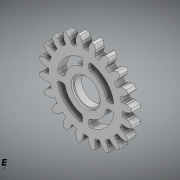
# Autodesk Inventor part: m2z20
Saved by Autodesk Inventor 2020 (Build 240168000, 168)
## iProperties
Created: 2019-12-19
Part Number: m2z20
Material: 一般
Document SubType Name: Modeling
Designer: hamaa
Density: 1 g/cm^3
Appearance: 既定
Author: hamaa
Autodesk Inventor part; units mm, degrees
(part 1 of 2)
ref_plane "YZ Plane" through (0, 0, 0) normal (1, 0, 0) x (0, 1, 0)
ref_plane "XZ Plane" through (0, 0, 0) normal (0, 1, 0) x (-1, 0, 0)
ref_plane "XY Plane" through (0, 0, 0) normal (0, 0, 1) x (1, 0, 0)
sketch "スケッチ1" plane through (0, 0, 0) normal (0, 0, 1) x (1, 0, 0)
  arc A0 (149.7476, 124.0441) -> (149.6952, 123.7559) centre (151.6276, 123.5535) ccw
  arc A1 (150.1104, 125.0278) -> (149.7476, 124.0441) centre (154.9305, 122.6916) ccw
  arc A2 (151.2536, 126.8271) -> (150.1104, 125.0278) centre (158.4906, 120.9661) ccw
  arc A3 (143.8017, 123.4975) -> (143.8409, 123.2073) centre (145.7412, 123.6119) ccw
  arc A4 (143.8427, 124.5452) -> (143.8017, 123.4975) centre (149.1488, 123.8129) ccw
  arc A5 (144.3739, 126.6097) -> (143.8427, 124.5452) centre (153.0679, 123.272) ccw
  arc A6 (138.3156, 121.1404) -> (138.4426, 120.8764) centre (140.1248, 121.8485) ccw
  arc A7 (138.0309, 122.1494) -> (138.3156, 121.1404) centre (143.3036, 123.0926) ccw
  arc A8 (137.8981, 124.2771) -> (138.0309, 122.1494) centre (147.198, 123.7893) ccw
  arc A9 (133.8264, 117.2033) -> (134.0288, 116.9915) centre (135.3283, 118.4358) ccw
  arc A10 (133.2438, 118.0749) -> (133.8264, 117.2033) centre (137.967, 120.6013) ccw
  arc A11 (132.4601, 120.0574) -> (133.2438, 118.0749) centre (141.4555, 122.4673) ccw
  arc A12 (130.7736, 112.0716) -> (131.0315, 111.9328) centre (131.8211, 113.708) ccw
  arc A13 (129.9502, 112.7206) -> (130.7736, 112.0716) centre (133.6615, 116.5829) ccw
  arc A14 (128.5922, 114.3639) -> (129.9502, 112.7206) centre (136.4027, 119.4356) ccw
  arc A15 (129.456, 106.2478) -> (129.7442, 106.1954) centre (129.9466, 108.1277) ccw
  arc A16 (128.4723, 106.6105) -> (129.456, 106.2478) centre (130.8085, 111.4307) ccw
  arc A17 (126.673, 107.7538) -> (128.4723, 106.6105) centre (132.5339, 114.9908) ccw
  arc A18 (130.0025, 100.3018) -> (130.2928, 100.341) centre (129.8882, 102.2413) ccw
  arc A19 (128.9549, 100.3428) -> (130.0025, 100.3018) centre (129.6872, 105.649) ccw
  arc A20 (126.8903, 100.8741) -> (128.9549, 100.3428) centre (130.2281, 109.568) ccw
  arc A21 (132.3597, 94.8158) -> (132.6237, 94.9428) centre (131.6516, 96.625) ccw
  arc A22 (131.3507, 94.531) -> (132.3597, 94.8158) centre (130.4075, 99.8038) ccw
  arc A23 (129.223, 94.3983) -> (131.3507, 94.531) centre (129.7108, 103.6981) ccw
  arc A24 (136.2968, 90.3266) -> (136.5086, 90.529) centre (135.0643, 91.8285) ccw
  arc A25 (135.4252, 89.744) -> (136.2968, 90.3266) centre (132.8988, 94.4672) ccw
  arc A26 (133.4426, 88.9603) -> (135.4252, 89.744) centre (131.0328, 97.9557) ccw
  arc A27 (141.4285, 87.2738) -> (141.5673, 87.5317) centre (139.7921, 88.3213) ccw
  arc A28 (140.7795, 86.4504) -> (141.4285, 87.2738) centre (136.9172, 90.1617) ccw
  arc A29 (139.1362, 85.0923) -> (140.7795, 86.4504) centre (134.0645, 92.9028) ccw
  arc A30 (147.2523, 85.9562) -> (147.3047, 86.2444) centre (145.3724, 86.4467) ccw
  arc A31 (146.8896, 84.9725) -> (147.2523, 85.9562) centre (142.0694, 87.3087) ccw
  arc A32 (145.7463, 83.1731) -> (146.8896, 84.9725) centre (138.5093, 89.0341) ccw
  arc A33 (153.1983, 86.5027) -> (153.159, 86.793) centre (151.2588, 86.3883) ccw
  arc A34 (153.1573, 85.4551) -> (153.1983, 86.5027) centre (147.8511, 86.1874) ccw
  arc A35 (152.626, 83.3905) -> (153.1573, 85.4551) centre (143.9321, 86.7283) ccw
  arc A36 (158.6843, 88.8599) -> (158.5573, 89.1238) centre (156.8751, 88.1518) ccw
  arc A37 (158.9691, 87.8509) -> (158.6843, 88.8599) centre (153.6963, 86.9076) ccw
  arc A38 (159.1018, 85.7232) -> (158.9691, 87.8509) centre (149.8019, 86.211) ccw
  arc A39 (163.1735, 92.797) -> (162.9711, 93.0088) centre (161.6716, 91.5644) ccw
  arc A40 (163.7561, 91.9254) -> (163.1735, 92.797) centre (159.0329, 89.3989) ccw
  arc A41 (164.5398, 89.9428) -> (163.7561, 91.9254) centre (155.5444, 87.5329) ccw
  arc A42 (166.2263, 97.9286) -> (165.9684, 98.0675) centre (165.1788, 96.2923) ccw
  arc A43 (167.0497, 97.2797) -> (166.2263, 97.9286) centre (163.3384, 93.4173) ccw
  arc A44 (168.4077, 95.6364) -> (167.0497, 97.2797) centre (160.5973, 90.5647) ccw
  arc A45 (167.5439, 103.7525) -> (167.2557, 103.8049) centre (167.0533, 101.8725) ccw
  arc A46 (168.5276, 103.3897) -> (167.5439, 103.7525) centre (166.1914, 98.5696) ccw
  arc A47 (170.327, 102.2465) -> (168.5276, 103.3897) centre (164.466, 95.0095) ccw
  arc A48 (166.9974, 109.6984) -> (166.7071, 109.6592) centre (167.1118, 107.7589) ccw
  arc A49 (168.045, 109.6574) -> (166.9974, 109.6984) centre (167.3127, 104.3513) ccw
  arc A50 (170.1096, 109.1262) -> (168.045, 109.6574) centre (166.7718, 100.4322) ccw
  arc A51 (164.6402, 115.1845) -> (164.3763, 115.0575) centre (165.3483, 113.3753) ccw
  arc A52 (165.6492, 115.4692) -> (164.6402, 115.1845) centre (166.5924, 110.1965) ccw
  arc A53 (167.7769, 115.602) -> (165.6492, 115.4692) centre (167.2891, 106.3021) ccw
  arc A54 (160.7031, 119.6736) -> (160.4913, 119.4713) centre (161.9356, 118.1718) ccw
  arc A55 (161.5747, 120.2563) -> (160.7031, 119.6736) centre (164.1012, 115.533) ccw
  arc A56 (163.5573, 121.04) -> (161.5747, 120.2563) centre (165.9672, 112.0445) ccw
  arc A57 (155.5715, 122.7265) -> (155.4326, 122.4686) centre (157.2078, 121.679) ccw
  arc A58 (156.2204, 123.5499) -> (155.5715, 122.7265) centre (160.0827, 119.8386) ccw
  arc A59 (157.8637, 124.9079) -> (156.2204, 123.5499) centre (162.9354, 117.0974) ccw
  arc A60 (147.3047, 123.7559) -> (147.2523, 124.0441) centre (145.3724, 123.5535) ccw
  arc A61 (147.2523, 124.0441) -> (146.8896, 125.0278) centre (142.0694, 122.6916) ccw
  arc A62 (146.8896, 125.0278) -> (145.7463, 126.8271) centre (138.5093, 120.9661) ccw
  arc A63 (141.5673, 122.4686) -> (141.4285, 122.7265) centre (139.7921, 121.679) ccw
  arc A64 (141.4285, 122.7265) -> (140.7795, 123.5499) centre (136.9172, 119.8386) ccw
  arc A65 (140.7795, 123.5499) -> (139.1362, 124.9079) centre (134.0645, 117.0974) ccw
  arc A66 (136.5086, 119.4713) -> (136.2968, 119.6736) centre (135.0643, 118.1718) ccw
  arc A67 (136.2968, 119.6736) -> (135.4252, 120.2563) centre (132.8988, 115.533) ccw
  arc A68 (135.4252, 120.2563) -> (133.4426, 121.04) centre (131.0328, 112.0445) ccw
  arc A69 (132.6237, 115.0575) -> (132.3597, 115.1845) centre (131.6516, 113.3753) ccw
  arc A70 (132.3597, 115.1845) -> (131.3507, 115.4692) centre (130.4075, 110.1965) ccw
  arc A71 (131.3507, 115.4692) -> (129.223, 115.602) centre (129.7108, 106.3021) ccw
  arc A72 (130.2928, 109.6592) -> (130.0025, 109.6984) centre (129.8882, 107.7589) ccw
  arc A73 (130.0025, 109.6984) -> (128.9549, 109.6574) centre (129.6872, 104.3513) ccw
  arc A74 (128.9549, 109.6574) -> (126.8903, 109.1262) centre (130.2281, 100.4322) ccw
  arc A75 (129.7442, 103.8049) -> (129.456, 103.7525) centre (129.9466, 101.8725) ccw
  arc A76 (129.456, 103.7525) -> (128.4723, 103.3897) centre (130.8085, 98.5696) ccw
  arc A77 (128.4723, 103.3897) -> (126.673, 102.2465) centre (132.5339, 95.0095) ccw
  arc A78 (131.0315, 98.0675) -> (130.7736, 97.9286) centre (131.8211, 96.2923) ccw
  arc A79 (130.7736, 97.9286) -> (129.9502, 97.2797) centre (133.6615, 93.4173) ccw
  arc A80 (129.9502, 97.2797) -> (128.5922, 95.6364) centre (136.4027, 90.5647) ccw
  arc A81 (134.0288, 93.0088) -> (133.8264, 92.797) centre (135.3283, 91.5644) ccw
  arc A82 (133.8264, 92.797) -> (133.2438, 91.9254) centre (137.967, 89.3989) ccw
  arc A83 (133.2438, 91.9254) -> (132.4601, 89.9428) centre (141.4555, 87.5329) ccw
  arc A84 (138.4426, 89.1238) -> (138.3156, 88.8599) centre (140.1248, 88.1518) ccw
  arc A85 (138.3156, 88.8599) -> (138.0309, 87.8509) centre (143.3036, 86.9076) ccw
  arc A86 (138.0309, 87.8509) -> (137.8981, 85.7232) centre (147.198, 86.211) ccw
  arc A87 (143.8409, 86.793) -> (143.8017, 86.5027) centre (145.7412, 86.3883) ccw
  arc A88 (143.8017, 86.5027) -> (143.8427, 85.4551) centre (149.1488, 86.1874) ccw
  arc A89 (143.8427, 85.4551) -> (144.3739, 83.3905) centre (153.0679, 86.7283) ccw
  arc A90 (149.6952, 86.2444) -> (149.7476, 85.9562) centre (151.6276, 86.4467) ccw
  arc A91 (149.7476, 85.9562) -> (150.1104, 84.9725) centre (154.9305, 87.3087) ccw
  arc A92 (150.1104, 84.9725) -> (151.2536, 83.1731) centre (158.4906, 89.0341) ccw
  arc A93 (155.4326, 87.5317) -> (155.5715, 87.2738) centre (157.2078, 88.3213) ccw
  arc A94 (155.5715, 87.2738) -> (156.2204, 86.4504) centre (160.0827, 90.1617) ccw
  arc A95 (156.2204, 86.4504) -> (157.8637, 85.0923) centre (162.9354, 92.9028) ccw
  arc A96 (160.4913, 90.529) -> (160.7031, 90.3266) centre (161.9356, 91.8285) ccw
  arc A97 (160.7031, 90.3266) -> (161.5747, 89.744) centre (164.1012, 94.4672) ccw
  arc A98 (161.5747, 89.744) -> (163.5573, 88.9603) centre (165.9672, 97.9557) ccw
  arc A99 (164.3763, 94.9428) -> (164.6402, 94.8158) centre (165.3483, 96.625) ccw
  arc A100 (164.6402, 94.8158) -> (165.6492, 94.531) centre (166.5924, 99.8038) ccw
  arc A101 (165.6492, 94.531) -> (167.7769, 94.3983) centre (167.2891, 103.6981) ccw
  arc A102 (166.7071, 100.341) -> (166.9974, 100.3018) centre (167.1118, 102.2413) ccw
  arc A103 (166.9974, 100.3018) -> (168.045, 100.3428) centre (167.3127, 105.649) ccw
  arc A104 (168.045, 100.3428) -> (170.1096, 100.8741) centre (166.7718, 109.568) ccw
  arc A105 (167.2557, 106.1954) -> (167.5439, 106.2478) centre (167.0533, 108.1277) ccw
  arc A106 (167.5439, 106.2478) -> (168.5276, 106.6105) centre (166.1914, 111.4307) ccw
  arc A107 (168.5276, 106.6105) -> (170.327, 107.7538) centre (164.466, 114.9908) ccw
  arc A108 (165.9684, 111.9328) -> (166.2263, 112.0716) centre (165.1788, 113.708) ccw
  arc A109 (166.2263, 112.0716) -> (167.0497, 112.7206) centre (163.3384, 116.5829) ccw
  arc A110 (167.0497, 112.7206) -> (168.4077, 114.3639) centre (160.5973, 119.4356) ccw
  arc A111 (162.9711, 116.9915) -> (163.1735, 117.2033) centre (161.6716, 118.4358) ccw
  arc A112 (163.1735, 117.2033) -> (163.7561, 118.0749) centre (159.0329, 120.6013) ccw
  arc A113 (163.7561, 118.0749) -> (164.5398, 120.0574) centre (155.5444, 122.4673) ccw
  arc A114 (158.5573, 120.8764) -> (158.6843, 121.1404) centre (156.8751, 121.8485) ccw
  arc A115 (158.6843, 121.1404) -> (158.9691, 122.1494) centre (153.6963, 123.0926) ccw
  arc A116 (158.9691, 122.1494) -> (159.1018, 124.2771) centre (149.8019, 123.7893) ccw
  arc A117 (153.159, 123.2073) -> (153.1983, 123.4975) centre (151.2588, 123.6119) ccw
  arc A118 (153.1983, 123.4975) -> (153.1573, 124.5452) centre (147.8511, 123.8129) ccw
  arc A119 (153.1573, 124.5452) -> (152.626, 126.6097) centre (143.9321, 123.272) ccw
  arc A120 (149.613, 122.4647) -> (147.387, 122.4647) centre (148.5, 105.0001) ccw
  arc A121 (144.1616, 121.9539) -> (142.0446, 121.266) centre (148.5, 105.0001) ccw
  arc A122 (139.135, 119.7835) -> (137.3341, 118.4751) centre (148.5, 105.0001) ccw
  arc A123 (135.025, 116.166) -> (133.7166, 114.3651) centre (148.5, 105.0001) ccw
  arc A124 (132.2341, 111.4555) -> (131.5462, 109.3385) centre (148.5, 105.0001) ccw
  arc A125 (131.0354, 106.1131) -> (131.0354, 103.8871) centre (148.5, 105.0001) ccw
  arc A126 (131.5462, 100.6618) -> (132.2341, 98.5448) centre (148.5, 105.0001) ccw
  arc A127 (133.7166, 95.6351) -> (135.025, 93.8343) centre (148.5, 105.0001) ccw
  arc A128 (137.3341, 91.5252) -> (139.135, 90.2168) centre (148.5, 105.0001) ccw
  arc A129 (142.0446, 88.7343) -> (144.1616, 88.0464) centre (148.5, 105.0001) ccw
  arc A130 (147.387, 87.5356) -> (149.613, 87.5356) centre (148.5, 105.0001) ccw
  arc A131 (152.8383, 88.0464) -> (154.9553, 88.7343) centre (148.5, 105.0001) ccw
  arc A132 (157.8649, 90.2168) -> (159.6658, 91.5252) centre (148.5, 105.0001) ccw
  arc A133 (161.9749, 93.8343) -> (163.2833, 95.6351) centre (148.5, 105.0001) ccw
  arc A134 (164.7658, 98.5448) -> (165.4537, 100.6618) centre (148.5, 105.0001) ccw
  arc A135 (165.9645, 103.8871) -> (165.9645, 106.1131) centre (148.5, 105.0001) ccw
  arc A136 (165.4537, 109.3385) -> (164.7658, 111.4555) centre (148.5, 105.0001) ccw
  arc A137 (163.2833, 114.3651) -> (161.9749, 116.166) centre (148.5, 105.0001) ccw
  arc A138 (159.6658, 118.4751) -> (157.8649, 119.7835) centre (148.5, 105.0001) ccw
  arc A139 (154.9553, 121.266) -> (152.8383, 121.9539) centre (148.5, 105.0001) ccw
  arc A140 (145.7463, 126.8271) -> (144.3739, 126.6097) centre (148.5, 105.0001) ccw
  arc A141 (139.1362, 124.9079) -> (137.8981, 124.2771) centre (148.5, 105.0001) ccw
  arc A142 (133.4426, 121.04) -> (132.4601, 120.0574) centre (148.5, 105.0001) ccw
  arc A143 (129.223, 115.602) -> (128.5922, 114.3639) centre (148.5, 105.0001) ccw
  arc A144 (126.8903, 109.1262) -> (126.673, 107.7538) centre (148.5, 105.0001) ccw
  arc A145 (126.673, 102.2465) -> (126.8903, 100.8741) centre (148.5, 105.0001) ccw
  arc A146 (128.5922, 95.6364) -> (129.223, 94.3983) centre (148.5, 105.0001) ccw
  arc A147 (132.4601, 89.9428) -> (133.4426, 88.9603) centre (148.5, 105.0001) ccw
  arc A148 (137.8981, 85.7232) -> (139.1362, 85.0923) centre (148.5, 105.0001) ccw
  arc A149 (144.3739, 83.3905) -> (145.7463, 83.1731) centre (148.5, 105.0001) ccw
  arc A150 (151.2536, 83.1731) -> (152.626, 83.3905) centre (148.5, 105.0001) ccw
  arc A151 (157.8637, 85.0923) -> (159.1018, 85.7232) centre (148.5, 105.0001) ccw
  arc A152 (163.5573, 88.9603) -> (164.5398, 89.9428) centre (148.5, 105.0001) ccw
  arc A153 (167.7769, 94.3983) -> (168.4077, 95.6364) centre (148.5, 105.0001) ccw
  arc A154 (170.1096, 100.8741) -> (170.327, 102.2465) centre (148.5, 105.0001) ccw
  arc A155 (170.327, 107.7538) -> (170.1096, 109.1262) centre (148.5, 105.0001) ccw
  arc A156 (168.4077, 114.3639) -> (167.7769, 115.602) centre (148.5, 105.0001) ccw
  arc A157 (164.5398, 120.0574) -> (163.5573, 121.04) centre (148.5, 105.0001) ccw
  arc A158 (159.1018, 124.2771) -> (157.8637, 124.9079) centre (148.5, 105.0001) ccw
  arc A159 (152.626, 126.6097) -> (151.2536, 126.8271) centre (148.5, 105.0001) ccw
  line L0 (149.613, 122.4647) -> (149.6952, 123.7559)
  line L1 (144.1616, 121.9539) -> (143.8409, 123.2073)
  line L2 (139.135, 119.7835) -> (138.4426, 120.8764)
  line L3 (135.025, 116.166) -> (134.0288, 116.9915)
  line L4 (132.2341, 111.4555) -> (131.0315, 111.9328)
  line L5 (131.0354, 106.1131) -> (129.7442, 106.1954)
  line L6 (131.5462, 100.6618) -> (130.2928, 100.341)
  line L7 (133.7166, 95.6351) -> (132.6237, 94.9428)
  line L8 (137.3341, 91.5252) -> (136.5086, 90.529)
  line L9 (142.0446, 88.7343) -> (141.5673, 87.5317)
  line L10 (147.387, 87.5356) -> (147.3047, 86.2444)
  line L11 (152.8383, 88.0464) -> (153.159, 86.793)
  line L12 (157.8649, 90.2168) -> (158.5573, 89.1238)
  line L13 (161.9749, 93.8343) -> (162.9711, 93.0088)
  line L14 (164.7658, 98.5448) -> (165.9684, 98.0675)
  line L15 (165.9645, 103.8871) -> (167.2557, 103.8049)
  line L16 (165.4537, 109.3385) -> (166.7071, 109.6592)
  line L17 (163.2833, 114.3651) -> (164.3763, 115.0575)
  line L18 (159.6658, 118.4751) -> (160.4913, 119.4713)
  line L19 (154.9553, 121.266) -> (155.4326, 122.4686)
  line L20 (147.387, 122.4647) -> (147.3047, 123.7559)
  line L21 (142.0446, 121.266) -> (141.5673, 122.4686)
  line L22 (137.3341, 118.4751) -> (136.5086, 119.4713)
  line L23 (133.7166, 114.3651) -> (132.6237, 115.0575)
  line L24 (131.5462, 109.3385) -> (130.2928, 109.6592)
  line L25 (131.0354, 103.8871) -> (129.7442, 103.8049)
  line L26 (132.2341, 98.5448) -> (131.0315, 98.0675)
  line L27 (135.025, 93.8343) -> (134.0288, 93.0088)
  line L28 (139.135, 90.2168) -> (138.4426, 89.1238)
  line L29 (144.1616, 88.0464) -> (143.8409, 86.793)
  line L30 (149.613, 87.5356) -> (149.6952, 86.2444)
  line L31 (154.9553, 88.7343) -> (155.4326, 87.5317)
  line L32 (159.6658, 91.5252) -> (160.4913, 90.529)
  line L33 (163.2833, 95.6351) -> (164.3763, 94.9428)
  line L34 (165.4537, 100.6618) -> (166.7071, 100.341)
  line L35 (165.9645, 106.1131) -> (167.2557, 106.1954)
  line L36 (164.7658, 111.4555) -> (165.9684, 111.9328)
  line L37 (161.9749, 116.166) -> (162.9711, 116.9915)
  line L38 (157.8649, 119.7835) -> (158.5573, 120.8764)
  line L39 (152.8383, 121.9539) -> (153.159, 123.2073)
  line L40 (124.5, 105) -> (172.5, 105)
  line L41 (148.5, 81) -> (148.5, 129)
  line L42 (190.5, 127.0001) -> (260.5, 127.0001)
  line L43 (190.5, 119.0001) -> (260.5, 119.0001)
  line L44 (190.5, 111.0001) -> (260.5, 111.0001)
  line L45 (190.5, 103.0001) -> (260.5, 103.0001)
  line L46 (190.5, 95.0001) -> (260.5, 95.0001)
  line L47 (190.5, 87.0001) -> (260.5, 87.0001)
  line L48 (190.5, 79.0001) -> (260.5, 79.0001)
  line L49 (190.5, 71.0001) -> (260.5, 71.0001)
  line L50 (190.5, 63.0001) -> (260.5, 63.0001)
  line L51 (190.5, 55.0001) -> (260.5, 55.0001)
  line L52 (190.5, 47.0001) -> (260.5, 47.0001)
  line L53 (190.5, 39.0001) -> (260.5, 39.0001)
  line L54 (190.5, 31.0001) -> (260.5, 31.0001)
  line L55 (190.5, 127.0001) -> (190.5, 31.0001)
  line L56 (260.5, 127.0001) -> (260.5, 31.0001)
  line L57 (225.5, 119.0001) -> (225.5, 31.0001)
  point P0 (0, 0)
  point P1 (196.5, 121)
  point P2 (199, 113)
  point P3 (199, 105)
  point P4 (196.5, 97)
  point P5 (199, 89)
  point P6 (194, 81)
  point P7 (196.5, 73)
  point P8 (196.5, 65)
  point P9 (196.5, 57)
  point P10 (199, 49)
  point P11 (199, 41)
  point P12 (196.5, 33)
  point P13 (226.5, 113)
  point P14 (241.5, 105)
  point P15 (242.75, 97)
  point P16 (239, 89)
  point P17 (241.5, 81)
  point P18 (235.25, 73)
  point P19 (241.5, 65)
  point P20 (241.5, 57)
  point P21 (236.5, 49)
  point P22 (244, 41)
  point P23 (244, 33)
  point P24 (149.5, 142.5)
  point P25 (149.5, 136.5)
  point P26 (165.6875, 142.5)
  point P27 (168.875, 136.5)
  constraints: 240 point on circle, 120 centre point, 117 equal radius, 112 end point, 80 tangent, 33 parallel, 22 horizontal, 12 perpendicular, 2 horizontal alignment, 2 midpoint, 2 vertical alignment, 171 other
extrude "押し出し1" add sketch "スケッチ1" along normal blind 4 contours A1 A2 A159 A119 A118 A117 L39 A139 L19 A57 A58 A59 A158 A116 A115 A114 L38 A138 L18 A54 A55 A56 A157 A113 A112 A111 L37 A137 L17 A51 A52 A53 A156 A110 A109 A108 L36 A136 L16 A48 A49 A50 A155 A107 A106 A105 L35 A135 L40 L41 A120 L0 A0 | L41 L40 A125 L5 A15 A16 A17 A144 A74 A73 A72 L24 A124 L4 A12 A13 A14 A143 A71 A70 A69 L23 A123 L3 A9 A10 A11 A142 A68 A67 A66 L22 A122 L2 A6 A7 A8 A141 A65 A64 A63 L21 A121 L1 A3 A4 A5 A140 A62 A61 A60 L20 A120 | L41 A130 L10 A30 A31 A32 A149 A89 A88 A87 L29 A129 L9 A27 A28 A29 A148 A86 A85 A84 L28 A128 L8 A24 A25 A26 A147 A83 A82 A81 L27 A127 L7 A21 A22 A23 A146 A80 A79 A78 L26 A126 L6 A18 A19 A20 A145 A77 A76 A75 L25 A125 L40 | L40 A135 L15 A45 A46 A47 A154 A104 A103 A102 L34 A134 L14 A42 A43 A44 A153 A101 A100 A99 L33 A133 L13 A39 A40 A41 A152 A98 A97 A96 L32 A132 L12 A36 A37 A38 A151 A95 A94 A93 L31 A131 L11 A33 A34 A35 A150 A92 A91 A90 L30 A130 L41
sketch "スケッチ2" plane through (0, 0, 4) normal (0, 0, 1) x (1, 0, 0)
  arc A0 (157.8649, 90.2168) -> (159.6658, 91.5252) centre (148.5, 105.0001) ccw projected
  line L0 (159.6658, 91.5252) -> (160.4913, 90.529) projected
  arc A1 (160.4913, 90.529) -> (160.7031, 90.3266) centre (161.9356, 91.8285) ccw projected
  arc A2 (160.7031, 90.3266) -> (161.5747, 89.744) centre (164.1012, 94.4672) ccw projected
  arc A3 (161.5747, 89.744) -> (163.5573, 88.9603) centre (165.9672, 97.9557) ccw projected
  arc A4 (163.5573, 88.9603) -> (164.5398, 89.9428) centre (148.5, 105.0001) ccw projected
  arc A5 (164.5398, 89.9428) -> (163.7561, 91.9254) centre (155.5444, 87.5329) ccw projected
  arc A6 (163.7561, 91.9254) -> (163.1735, 92.797) centre (159.0329, 89.3989) ccw projected
  arc A7 (163.1735, 92.797) -> (162.9711, 93.0088) centre (161.6716, 91.5644) ccw projected
  line L1 (162.9711, 93.0088) -> (161.9749, 93.8343) projected
  arc A8 (161.9749, 93.8343) -> (163.2833, 95.6351) centre (148.5, 105.0001) ccw projected
  line L2 (163.2833, 95.6351) -> (164.3763, 94.9428) projected
  arc A9 (164.3763, 94.9428) -> (164.6402, 94.8158) centre (165.3483, 96.625) ccw projected
  arc A10 (164.6402, 94.8158) -> (165.6492, 94.531) centre (166.5924, 99.8038) ccw projected
  arc A11 (165.6492, 94.531) -> (167.7769, 94.3983) centre (167.2891, 103.6981) ccw projected
  arc A12 (167.7769, 94.3983) -> (168.4077, 95.6364) centre (148.5, 105.0001) ccw projected
  arc A13 (168.4077, 95.6364) -> (167.0497, 97.2797) centre (160.5973, 90.5647) ccw projected
  arc A14 (167.0497, 97.2797) -> (166.2263, 97.9286) centre (163.3384, 93.4173) ccw projected
  arc A15 (166.2263, 97.9286) -> (165.9684, 98.0675) centre (165.1788, 96.2923) ccw projected
  line L3 (165.9684, 98.0675) -> (164.7658, 98.5448) projected
  arc A16 (164.7658, 98.5448) -> (165.4537, 100.6618) centre (148.5, 105.0001) ccw projected
  line L4 (165.4537, 100.6618) -> (166.7071, 100.341) projected
  arc A17 (166.7071, 100.341) -> (166.9974, 100.3018) centre (167.1118, 102.2413) ccw projected
  arc A18 (166.9974, 100.3018) -> (168.045, 100.3428) centre (167.3127, 105.649) ccw projected
  arc A19 (168.045, 100.3428) -> (170.1096, 100.8741) centre (166.7718, 109.568) ccw projected
  arc A20 (170.1096, 100.8741) -> (170.327, 102.2465) centre (148.5, 105.0001) ccw projected
  arc A21 (170.327, 102.2465) -> (168.5276, 103.3897) centre (164.466, 95.0095) ccw projected
  arc A22 (168.5276, 103.3897) -> (167.5439, 103.7525) centre (166.1914, 98.5696) ccw projected
  arc A23 (167.5439, 103.7525) -> (167.2557, 103.8049) centre (167.0533, 101.8725) ccw projected
  line L5 (167.2557, 103.8049) -> (165.9645, 103.8871) projected
  arc A24 (165.9645, 103.8871) -> (165.9645, 106.1131) centre (148.5, 105.0001) ccw projected
  line L6 (165.9645, 106.1131) -> (167.2557, 106.1954) projected
  arc A25 (167.2557, 106.1954) -> (167.5439, 106.2478) centre (167.0533, 108.1277) ccw projected
  arc A26 (167.5439, 106.2478) -> (168.5276, 106.6105) centre (166.1914, 111.4307) ccw projected
  arc A27 (168.5276, 106.6105) -> (170.327, 107.7538) centre (164.466, 114.9908) ccw projected
  arc A28 (170.327, 107.7538) -> (170.1096, 109.1262) centre (148.5, 105.0001) ccw projected
  arc A29 (170.1096, 109.1262) -> (168.045, 109.6574) centre (166.7718, 100.4322) ccw projected
  arc A30 (168.045, 109.6574) -> (166.9974, 109.6984) centre (167.3127, 104.3513) ccw projected
  arc A31 (166.9974, 109.6984) -> (166.7071, 109.6592) centre (167.1118, 107.7589) ccw projected
  line L7 (166.7071, 109.6592) -> (165.4537, 109.3385) projected
  arc A32 (165.4537, 109.3385) -> (164.7658, 111.4555) centre (148.5, 105.0001) ccw projected
  line L8 (164.7658, 111.4555) -> (165.9684, 111.9328) projected
  arc A33 (165.9684, 111.9328) -> (166.2263, 112.0716) centre (165.1788, 113.708) ccw projected
  arc A34 (166.2263, 112.0716) -> (167.0497, 112.7206) centre (163.3384, 116.5829) ccw projected
  arc A35 (167.0497, 112.7206) -> (168.4077, 114.3639) centre (160.5973, 119.4356) ccw projected
  arc A36 (168.4077, 114.3639) -> (167.7769, 115.602) centre (148.5, 105.0001) ccw projected
  arc A37 (167.7769, 115.602) -> (165.6492, 115.4692) centre (167.2891, 106.3021) ccw projected
  arc A38 (165.6492, 115.4692) -> (164.6402, 115.1845) centre (166.5924, 110.1965) ccw projected
  arc A39 (164.6402, 115.1845) -> (164.3763, 115.0575) centre (165.3483, 113.3753) ccw projected
  line L9 (164.3763, 115.0575) -> (163.2833, 114.3651) projected
  arc A40 (163.2833, 114.3651) -> (161.9749, 116.166) centre (148.5, 105.0001) ccw projected
  line L10 (161.9749, 116.166) -> (162.9711, 116.9915) projected
  arc A41 (162.9711, 116.9915) -> (163.1735, 117.2033) centre (161.6716, 118.4358) ccw projected
  arc A42 (163.1735, 117.2033) -> (163.7561, 118.0749) centre (159.0329, 120.6013) ccw projected
  arc A43 (163.7561, 118.0749) -> (164.5398, 120.0574) centre (155.5444, 122.4673) ccw projected
  arc A44 (164.5398, 120.0574) -> (163.5573, 121.04) centre (148.5, 105.0001) ccw projected
  arc A45 (163.5573, 121.04) -> (161.5747, 120.2563) centre (165.9672, 112.0445) ccw projected
  arc A46 (161.5747, 120.2563) -> (160.7031, 119.6736) centre (164.1012, 115.533) ccw projected
  arc A47 (160.7031, 119.6736) -> (160.4913, 119.4713) centre (161.9356, 118.1718) ccw projected
  line L11 (160.4913, 119.4713) -> (159.6658, 118.4751) projected
  arc A48 (159.6658, 118.4751) -> (157.8649, 119.7835) centre (148.5, 105.0001) ccw projected
  line L12 (157.8649, 119.7835) -> (158.5573, 120.8764) projected
  arc A49 (158.5573, 120.8764) -> (158.6843, 121.1404) centre (156.8751, 121.8485) ccw projected
  arc A50 (158.6843, 121.1404) -> (158.9691, 122.1494) centre (153.6963, 123.0926) ccw projected
  arc A51 (158.9691, 122.1494) -> (159.1018, 124.2771) centre (149.8019, 123.7893) ccw projected
  arc A52 (159.1018, 124.2771) -> (157.8637, 124.9079) centre (148.5, 105.0001) ccw projected
  arc A53 (157.8637, 124.9079) -> (156.2204, 123.5499) centre (162.9354, 117.0974) ccw projected
  arc A54 (156.2204, 123.5499) -> (155.5715, 122.7265) centre (160.0827, 119.8386) ccw projected
  arc A55 (155.5715, 122.7265) -> (155.4326, 122.4686) centre (157.2078, 121.679) ccw projected
  line L13 (155.4326, 122.4686) -> (154.9553, 121.266) projected
  arc A56 (154.9553, 121.266) -> (152.8383, 121.9539) centre (148.5, 105.0001) ccw projected
  line L14 (152.8383, 121.9539) -> (153.159, 123.2073) projected
  arc A57 (153.159, 123.2073) -> (153.1983, 123.4975) centre (151.2588, 123.6119) ccw projected
  arc A58 (153.1983, 123.4975) -> (153.1573, 124.5452) centre (147.8511, 123.8129) ccw projected
  arc A59 (153.1573, 124.5452) -> (152.626, 126.6097) centre (143.9321, 123.272) ccw projected
  arc A60 (152.626, 126.6097) -> (151.2536, 126.8271) centre (148.5, 105.0001) ccw projected
  arc A61 (151.2536, 126.8271) -> (150.1104, 125.0278) centre (158.4906, 120.9661) ccw projected
  arc A62 (150.1104, 125.0278) -> (149.7476, 124.0441) centre (154.9305, 122.6916) ccw projected
  arc A63 (149.7476, 124.0441) -> (149.6952, 123.7559) centre (151.6276, 123.5535) ccw projected
  line L15 (149.6952, 123.7559) -> (149.613, 122.4647) projected
  arc A64 (149.613, 122.4647) -> (147.387, 122.4647) centre (148.5, 105.0001) ccw projected
  line L16 (147.387, 122.4647) -> (147.3047, 123.7559) projected
  arc A65 (147.3047, 123.7559) -> (147.2523, 124.0441) centre (145.3724, 123.5535) ccw projected
  arc A66 (147.2523, 124.0441) -> (146.8896, 125.0278) centre (142.0694, 122.6916) ccw projected
  arc A67 (146.8896, 125.0278) -> (145.7463, 126.8271) centre (138.5093, 120.9661) ccw projected
  arc A68 (145.7463, 126.8271) -> (144.3739, 126.6097) centre (148.5, 105.0001) ccw projected
  arc A69 (144.3739, 126.6097) -> (143.8427, 124.5452) centre (153.0679, 123.272) ccw projected
  arc A70 (143.8427, 124.5452) -> (143.8017, 123.4975) centre (149.1488, 123.8129) ccw projected
  arc A71 (143.8017, 123.4975) -> (143.8409, 123.2073) centre (145.7412, 123.6119) ccw projected
  line L17 (143.8409, 123.2073) -> (144.1616, 121.9539) projected
  arc A72 (144.1616, 121.9539) -> (142.0446, 121.266) centre (148.5, 105.0001) ccw projected
  line L18 (142.0446, 121.266) -> (141.5673, 122.4686) projected
  arc A73 (141.5673, 122.4686) -> (141.4285, 122.7265) centre (139.7921, 121.679) ccw projected
  arc A74 (141.4285, 122.7265) -> (140.7795, 123.5499) centre (136.9172, 119.8386) ccw projected
  arc A75 (140.7795, 123.5499) -> (139.1362, 124.9079) centre (134.0645, 117.0974) ccw projected
  arc A76 (139.1362, 124.9079) -> (137.8981, 124.2771) centre (148.5, 105.0001) ccw projected
  arc A77 (137.8981, 124.2771) -> (138.0309, 122.1494) centre (147.198, 123.7893) ccw projected
  arc A78 (138.0309, 122.1494) -> (138.3156, 121.1404) centre (143.3036, 123.0926) ccw projected
  arc A79 (138.3156, 121.1404) -> (138.4426, 120.8764) centre (140.1248, 121.8485) ccw projected
  line L19 (138.4426, 120.8764) -> (139.135, 119.7835) projected
  arc A80 (139.135, 119.7835) -> (137.3341, 118.4751) centre (148.5, 105.0001) ccw projected
  line L20 (137.3341, 118.4751) -> (136.5086, 119.4713) projected
  arc A81 (136.5086, 119.4713) -> (136.2968, 119.6736) centre (135.0643, 118.1718) ccw projected
  arc A82 (136.2968, 119.6736) -> (135.4252, 120.2563) centre (132.8988, 115.533) ccw projected
  arc A83 (135.4252, 120.2563) -> (133.4426, 121.04) centre (131.0328, 112.0445) ccw projected
  arc A84 (133.4426, 121.04) -> (132.4601, 120.0574) centre (148.5, 105.0001) ccw projected
  arc A85 (132.4601, 120.0574) -> (133.2438, 118.0749) centre (141.4555, 122.4673) ccw projected
  arc A86 (133.2438, 118.0749) -> (133.8264, 117.2033) centre (137.967, 120.6013) ccw projected
  arc A87 (133.8264, 117.2033) -> (134.0288, 116.9915) centre (135.3283, 118.4358) ccw projected
  line L21 (134.0288, 116.9915) -> (135.025, 116.166) projected
  arc A88 (135.025, 116.166) -> (133.7166, 114.3651) centre (148.5, 105.0001) ccw projected
  line L22 (133.7166, 114.3651) -> (132.6237, 115.0575) projected
  arc A89 (132.6237, 115.0575) -> (132.3597, 115.1845) centre (131.6516, 113.3753) ccw projected
  arc A90 (132.3597, 115.1845) -> (131.3507, 115.4692) centre (130.4075, 110.1965) ccw projected
  arc A91 (131.3507, 115.4692) -> (129.223, 115.602) centre (129.7108, 106.3021) ccw projected
  arc A92 (129.223, 115.602) -> (128.5922, 114.3639) centre (148.5, 105.0001) ccw projected
  arc A93 (128.5922, 114.3639) -> (129.9502, 112.7206) centre (136.4027, 119.4356) ccw projected
  arc A94 (129.9502, 112.7206) -> (130.7736, 112.0716) centre (133.6615, 116.5829) ccw projected
  arc A95 (130.7736, 112.0716) -> (131.0315, 111.9328) centre (131.8211, 113.708) ccw projected
  line L23 (131.0315, 111.9328) -> (132.2341, 111.4555) projected
  arc A96 (132.2341, 111.4555) -> (131.5462, 109.3385) centre (148.5, 105.0001) ccw projected
  line L24 (131.5462, 109.3385) -> (130.2928, 109.6592) projected
  arc A97 (130.2928, 109.6592) -> (130.0025, 109.6984) centre (129.8882, 107.7589) ccw projected
  arc A98 (130.0025, 109.6984) -> (128.9549, 109.6574) centre (129.6872, 104.3513) ccw projected
  arc A99 (128.9549, 109.6574) -> (126.8903, 109.1262) centre (130.2281, 100.4322) ccw projected
  arc A100 (126.8903, 109.1262) -> (126.673, 107.7538) centre (148.5, 105.0001) ccw projected
  arc A101 (126.673, 107.7538) -> (128.4723, 106.6105) centre (132.5339, 114.9908) ccw projected
  arc A102 (128.4723, 106.6105) -> (129.456, 106.2478) centre (130.8085, 111.4307) ccw projected
  arc A103 (129.456, 106.2478) -> (129.7442, 106.1954) centre (129.9466, 108.1277) ccw projected
  line L25 (129.7442, 106.1954) -> (131.0354, 106.1131) projected
  arc A104 (131.0354, 106.1131) -> (131.0354, 103.8871) centre (148.5, 105.0001) ccw projected
  line L26 (131.0354, 103.8871) -> (129.7442, 103.8049) projected
  arc A105 (129.7442, 103.8049) -> (129.456, 103.7525) centre (129.9466, 101.8725) ccw projected
  arc A106 (129.456, 103.7525) -> (128.4723, 103.3897) centre (130.8085, 98.5696) ccw projected
  arc A107 (128.4723, 103.3897) -> (126.673, 102.2465) centre (132.5339, 95.0095) ccw projected
  arc A108 (126.673, 102.2465) -> (126.8903, 100.8741) centre (148.5, 105.0001) ccw projected
  arc A109 (126.8903, 100.8741) -> (128.9549, 100.3428) centre (130.2281, 109.568) ccw projected
  arc A110 (128.9549, 100.3428) -> (130.0025, 100.3018) centre (129.6872, 105.649) ccw projected
  arc A111 (130.0025, 100.3018) -> (130.2928, 100.341) centre (129.8882, 102.2413) ccw projected
  line L27 (130.2928, 100.341) -> (131.5462, 100.6618) projected
  arc A112 (131.5462, 100.6618) -> (132.2341, 98.5448) centre (148.5, 105.0001) ccw projected
  line L28 (132.2341, 98.5448) -> (131.0315, 98.0675) projected
  arc A113 (131.0315, 98.0675) -> (130.7736, 97.9286) centre (131.8211, 96.2923) ccw projected
  arc A114 (130.7736, 97.9286) -> (129.9502, 97.2797) centre (133.6615, 93.4173) ccw projected
  arc A115 (129.9502, 97.2797) -> (128.5922, 95.6364) centre (136.4027, 90.5647) ccw projected
  arc A116 (128.5922, 95.6364) -> (129.223, 94.3983) centre (148.5, 105.0001) ccw projected
  arc A117 (129.223, 94.3983) -> (131.3507, 94.531) centre (129.7108, 103.6981) ccw projected
  arc A118 (131.3507, 94.531) -> (132.3597, 94.8158) centre (130.4075, 99.8038) ccw projected
  arc A119 (132.3597, 94.8158) -> (132.6237, 94.9428) centre (131.6516, 96.625) ccw projected
  line L29 (132.6237, 94.9428) -> (133.7166, 95.6351) projected
  arc A120 (133.7166, 95.6351) -> (135.025, 93.8343) centre (148.5, 105.0001) ccw projected
  line L30 (135.025, 93.8343) -> (134.0288, 93.0088) projected
  arc A121 (134.0288, 93.0088) -> (133.8264, 92.797) centre (135.3283, 91.5644) ccw projected
  arc A122 (133.8264, 92.797) -> (133.2438, 91.9254) centre (137.967, 89.3989) ccw projected
  arc A123 (133.2438, 91.9254) -> (132.4601, 89.9428) centre (141.4555, 87.5329) ccw projected
  arc A124 (132.4601, 89.9428) -> (133.4426, 88.9603) centre (148.5, 105.0001) ccw projected
  arc A125 (133.4426, 88.9603) -> (135.4252, 89.744) centre (131.0328, 97.9557) ccw projected
  arc A126 (135.4252, 89.744) -> (136.2968, 90.3266) centre (132.8988, 94.4672) ccw projected
  arc A127 (136.2968, 90.3266) -> (136.5086, 90.529) centre (135.0643, 91.8285) ccw projected
  line L31 (136.5086, 90.529) -> (137.3341, 91.5252) projected
  arc A128 (137.3341, 91.5252) -> (139.135, 90.2168) centre (148.5, 105.0001) ccw projected
  line L32 (139.135, 90.2168) -> (138.4426, 89.1238) projected
  arc A129 (138.4426, 89.1238) -> (138.3156, 88.8599) centre (140.1248, 88.1518) ccw projected
  arc A130 (138.3156, 88.8599) -> (138.0309, 87.8509) centre (143.3036, 86.9076) ccw projected
  arc A131 (138.0309, 87.8509) -> (137.8981, 85.7232) centre (147.198, 86.211) ccw projected
  arc A132 (137.8981, 85.7232) -> (139.1362, 85.0923) centre (148.5, 105.0001) ccw projected
  arc A133 (139.1362, 85.0923) -> (140.7795, 86.4504) centre (134.0645, 92.9028) ccw projected
  arc A134 (140.7795, 86.4504) -> (141.4285, 87.2738) centre (136.9172, 90.1617) ccw projected
  arc A135 (141.4285, 87.2738) -> (141.5673, 87.5317) centre (139.7921, 88.3213) ccw projected
  line L33 (141.5673, 87.5317) -> (142.0446, 88.7343) projected
  arc A136 (142.0446, 88.7343) -> (144.1616, 88.0464) centre (148.5, 105.0001) ccw projected
  line L34 (144.1616, 88.0464) -> (143.8409, 86.793) projected
  arc A137 (143.8409, 86.793) -> (143.8017, 86.5027) centre (145.7412, 86.3883) ccw projected
  arc A138 (143.8017, 86.5027) -> (143.8427, 85.4551) centre (149.1488, 86.1874) ccw projected
  arc A139 (143.8427, 85.4551) -> (144.3739, 83.3905) centre (153.0679, 86.7283) ccw projected
  arc A140 (144.3739, 83.3905) -> (145.7463, 83.1731) centre (148.5, 105.0001) ccw projected
  arc A141 (145.7463, 83.1731) -> (146.8896, 84.9725) centre (138.5093, 89.0341) ccw projected
  arc A142 (146.8896, 84.9725) -> (147.2523, 85.9562) centre (142.0694, 87.3087) ccw projected
  arc A143 (147.2523, 85.9562) -> (147.3047, 86.2444) centre (145.3724, 86.4467) ccw projected
  line L35 (147.3047, 86.2444) -> (147.387, 87.5356) projected
  arc A144 (147.387, 87.5356) -> (149.613, 87.5356) centre (148.5, 105.0001) ccw projected
  line L36 (149.613, 87.5356) -> (149.6952, 86.2444) projected
  arc A145 (149.6952, 86.2444) -> (149.7476, 85.9562) centre (151.6276, 86.4467) ccw projected
  arc A146 (149.7476, 85.9562) -> (150.1104, 84.9725) centre (154.9305, 87.3087) ccw projected
  arc A147 (150.1104, 84.9725) -> (151.2536, 83.1731) centre (158.4906, 89.0341) ccw projected
  arc A148 (151.2536, 83.1731) -> (152.626, 83.3905) centre (148.5, 105.0001) ccw projected
  arc A149 (152.626, 83.3905) -> (153.1573, 85.4551) centre (143.9321, 86.7283) ccw projected
  arc A150 (153.1573, 85.4551) -> (153.1983, 86.5027) centre (147.8511, 86.1874) ccw projected
  arc A151 (153.1983, 86.5027) -> (153.159, 86.793) centre (151.2588, 86.3883) ccw projected
  line L37 (153.159, 86.793) -> (152.8383, 88.0464) projected
  arc A152 (152.8383, 88.0464) -> (154.9553, 88.7343) centre (148.5, 105.0001) ccw projected
  line L38 (154.9553, 88.7343) -> (155.4326, 87.5317) projected
  arc A153 (155.4326, 87.5317) -> (155.5715, 87.2738) centre (157.2078, 88.3213) ccw projected
  arc A154 (155.5715, 87.2738) -> (156.2204, 86.4504) centre (160.0827, 90.1617) ccw projected
  arc A155 (156.2204, 86.4504) -> (157.8637, 85.0923) centre (162.9354, 92.9028) ccw projected
  arc A156 (157.8637, 85.0923) -> (159.1018, 85.7232) centre (148.5, 105.0001) ccw projected
  arc A157 (159.1018, 85.7232) -> (158.9691, 87.8509) centre (149.8019, 86.211) ccw projected
  arc A158 (158.9691, 87.8509) -> (158.6843, 88.8599) centre (153.6963, 86.9076) ccw projected
  arc A159 (158.6843, 88.8599) -> (158.5573, 89.1238) centre (156.8751, 88.1518) ccw projected
  line L39 (158.5573, 89.1238) -> (157.8649, 90.2168) projected
  circle A160 centre (148.5, 105.0001) radius 6
  circle A161 centre (148.5, 105.0001) radius 6.8
  point P0 (0, 0)
  dimension "d2" = 12
  dimension "d3" = 0.8
  constraints: 2 centre point, 1 coincident
  measures "d2" diameter of A160
  measures "d3" radial gap between concentric circles of A160 A161
extrude "押し出し2" cut sketch "スケッチ2" against normal blind 4 contours A160
extrude "押し出し3" cut sketch "スケッチ2" against normal blind 0.8 contours A161